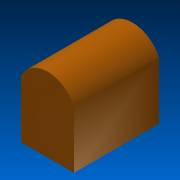
# Autodesk Inventor part: Omron SS-01GL2-E Microswitch Button
Saved by Autodesk Inventor 2013 (Build 170138000, 138)
## iProperties
Created: 2012-05-23
Material: ABS Plastic
Document SubType Name: Modeling
Designer: sdarley
Density: 1 g/cm^3
Project: Microswitch - Omron SS-01GL2-E
Description: Omron SS-01GL2-E Microswitch Button
Author: sdarley
Title: Omron SS-01GL2-E Microswitch Button
Revision Number: 1
Autodesk Inventor part; units mm, degrees
ref_plane "YZ Plane" through (0, 0, 0) normal (1, 0, 0) x (0, 1, 0)
ref_plane "XZ Plane" through (0, 0, 0) normal (0, 1, 0) x (-1, 0, 0)
ref_plane "XY Plane" through (0, 0, 0) normal (0, 0, 1) x (1, 0, 0)
sketch "Sketch1" plane through (0, 0, 0) normal (0, 1, 0) x (-1, 0, 0)
  line L0 (-1, 0) -> (1, 0)
  line L1 (1, 0) -> (1, 2.1583)
  line L2 (-1, 0) -> (-1, 2.1583)
  arc A0 (1, 2.1583) -> (-1, 2.1583) centre (0, 1.7) ccw
  line L3 (3.4698, 1.8) -> (-2.375, 1.8) projected
  point P0 (0, 0)
  point P1 (0, 0)
  dimension "d0" = 2
  dimension "d2" = 2.8
  dimension "d6" = 1.1
  constraints: 6 end point, 2 horizontal alignment, 2 point on circle, 1 centre point, 1 coincident, 1 horizontal, 1 midpoint, 1 parallel, 1 perpendicular
  measures "d0" distance of L0.start L0.end
  measures "d6" radius of A0
extrude "Extrusion1" add sketch "Sketch1" along normal mid plane 3.2
body "Solid1"
